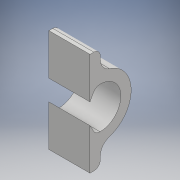
# Autodesk Inventor part: binding links
Saved by Autodesk Inventor 2017 (Build 210142000, 142)
## iProperties
Part Number: binding links
Material: Типовые
Document SubType Name: Modeling
Designer: TRENER
Density: 1 g/cm^3
Appearance: По умолчанию
Author: TRENER
Autodesk Inventor part; units mm, degrees
ref_plane "YZ Plane" through (0, 0, 0) normal (1, 0, 0) x (0, 1, 0)
ref_plane "XZ Plane" through (0, 0, 0) normal (0, 1, 0) x (-1, 0, 0)
ref_plane "XY Plane" through (0, 0, 0) normal (0, 0, 1) x (1, 0, 0)
sketch "Эскиз1" plane through (0, 0, 0) normal (1, 0, 0) x (0, 1, 0)
  circle A0 centre (0, 0) radius 4
  circle A1 centre (0, 0) radius 5
  line L0 (0, 5) -> (-2, 5)
  line L1 (-2, 5) -> (-2, 10)
  line L2 (-2, 10) -> (0, 10)
  line L3 (0, 10) -> (0, 5)
  line L4 (0, -5) -> (-2, -5)
  line L5 (-2, -5) -> (-2, -10)
  line L6 (-2, -10) -> (0, -10)
  line L7 (0, -10) -> (0, -5)
  line L8 (-2, 5) -> (-2, -5)
  line L9 (0, 5) -> (-2, 4.5826)
  line L10 (-2, -4.5826) -> (0, -5)
  line L11 (-2, 2) -> (-1, 3.873)
  line L12 (-2, -2) -> (-1, -3.873)
  line L13 (-1, -3.873) -> (-2, -3.873)
  line L14 (-1, 3.873) -> (-2, 3.873)
  dimension "d0" = 8
  dimension "d1" = 10
  dimension "d2" = 3
  dimension "d3" = 3
  constraints: 30 end point, 7 point on line, 6 point on circle, 4 parallel, 4 perpendicular, 2 centre point, 2 coincident, 2 horizontal
  measures "d0" diameter of A0
  measures "d1" diameter of A1
  measures "d2" distance from line of L0 L11.start
  measures "d3" distance from line of L4 L12.start
extrude "Выдавливание1" add sketch "Эскиз1" along normal blind 8 contours A0 L14 L8 L9 A1 L10 L13 | L11 L8 A0 | A0 L8 L14 | L13 L8 A0 | A0 L8 L12 | L8 L0 A1 | A1 L9 | L10 A1 | A1 L4 L8 | L0 L1 L2 L3 | L7 L6 L5 L4
fillet "Сопряжение2" radius 1.25 2 edges at (4, 0, 10) (4, 0, -10)
fillet "Сопряжение3" radius 1.5 2 edges at (4, -1, -3.873) (4, -1, 3.873)
sketch "Эскиз5" plane through (8, 0, 0) normal (1, 0, 0) x (0, 0, -1)
  circle A0 centre (0, 0) radius 5
  circle A1 centre (0, 0) radius 6
  line L0 (-5, 0) -> (-8.75, 0) projected
  line L1 (-6, 0) -> (-5, 0)
  arc A2 (5, 0) -> (-5, 0) centre (0, 0) ccw projected
  line L2 (-5, 0) -> (5, 0)
  line L3 (8.75, 0) -> (5, 0) projected
  line L4 (6, 0) -> (5, 0)
  dimension "d28" = 12
  constraints: 6 end point, 2 centre point, 2 coincident, 2 collinear, 2 point on circle, 1 horizontal, 1 point on line
  measures "d28" diameter of A1
extrude "Выдавливание5" add sketch "Эскиз5" against normal blind 8 contours A0 L0 A1 L3 picked at (-5.5601, 0.8775)
fillet "Сопряжение4" radius 2.5 2 edges at (4, 0, 6) (4, 0, -6)
